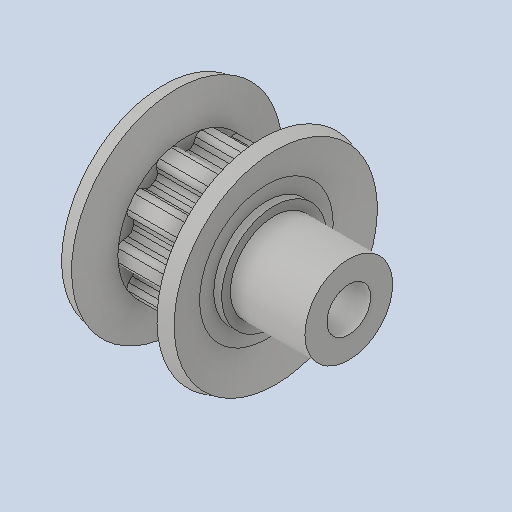
# Autodesk Inventor part: STP10XL025-B-H5_b
Saved by Autodesk Inventor 2024.1 (Build 281209000, 209)
## iProperties
Created: 2023-12-09
Part Number: STP10XL025-B-H5_b
Material: Generic
Catalog Web Link: www.cadenas.de
Description: ATP__XL025, ATP__XL031, ATP__ XL037, ATP__XL050, BTP__XL025, BTP__XL031, BTP__XL037, BTP__XL050, KTP__XL025, KTP__XL031, KTP__ XL037, KTP__XL050, NTP__XL025, NTP__XL031, NTP__ XL037, NTP__XL050, MTP__XL025, MTP__ XL037, MTP__XL050, MTPB__XL025, MTPB__ XL037, MTPB__XL050, MTPP__XL025, MTPP__ XL037, MTPP__XL050, STP__XL025, STP__XL031, STP__ XL037, STP__XL050, KATP__XL025, KATP__XL031, KATP__ XL037, KATP__XL050, KKTP__XL025, KKTP__XL031, KKTP__ XL037, KKTP__XL050_body-Timing Pulleys XL Type
Vendor: MISUMI
Document SubType Name: Modeling
Designer: psAdmin
Manufacturer: MISUMI
Mass: 3.12831 g
Surface Area: 27.7285 cm^2
Volume: 3.12831 cm^3
Density: 1 g/cm^3
Appearance: PSOLRGB-175-175-175
Category: PARTsolutions
Company: MISUMI
PSOL_IDENT_0: {$CADENAS_DATA/23d-libs/misumi/metric/51_timing_pulleys/mtp_xl/mtp_xl.prj},886 {VTYP=3D},{NB=STP10XL
PSOL_IDENT_1: 025-B-H5_b},{LINA=STP10XL025-B-H5},{NN=ATP__XL025, ATP__XL031, ATP__ XL037, ATP__XL050, BTP__XL025,
PSOL_IDENT_2: BTP__XL031, BTP__XL037, BTP__XL050, KTP__XL025, KTP__XL031, KTP__ XL037, KTP__XL050, NTP__XL025, NTP
PSOL_IDENT_3: __XL031, NTP__ XL037, NTP__XL050, MTP__XL025, MTP__ XL037, MTP__XL050, MTPB__XL025, MTPB__ XL037, MT
PSOL_IDENT_4: PB__XL050, MTPP__XL025, MTPP__ XL037, MTPP__XL050, STP__XL025, STP__XL031, STP__ XL037, STP__XL050,
PSOL_IDENT_5: KATP__XL025, KATP__XL031, KATP__ XL037, KATP__XL050, KKTP__XL025, KKTP__XL031, KKTP__ XL037, KKTP__X
PSOL_IDENT_6: L050_body},{DATE=06.01.2023 09:07:12},{GEOMDATE=06.01.2023 09:06:51},{VERSION=},{LINEID=290},{WBVAR=
PSOL_IDENT_7: MATP,ST,TNW,PS,SBS,DD,Z,J,Q,R,S,T,ALT1,ALT2,M,QSC,QFC,QTC,ALT3,K,KSC,KFC,KTC,ALT4,ZM,ZSC,ZFC,ZTC,ALT
PSOL_IDENT_8: 5,ALT6,ALT7,FC,ALT8,SRG,ALT9,BTC,TL,ALT10,TPC,ALT11,BC,ALT12,SLH,ALT13,BN},{WBNUMERIC=DD,Z,J,Q,R,S,T
PSOL_IDENT_9: ,QSC,QFC,QTC,K,KSC,KFC,KTC,ZSC,ZFC,ZTC,FC,SRG,BTC,TL,BC,SLH,BN}  {NB=STP10XL025-B-H5_b},{LINA=STP10X
PSOL_IDENT_10: L025-B-H5},{KT=DUMMY},{PN=STP10XL025-B-H5},{TYPE=STP},{MATP=SUS304},{MATPALG= 'A2017','Aluminum Allo
PSOL_IDENT_11: y 2000 series','S45C','1045 Carbon Steel Equivalent','SUS304','SUS304', 'A6000', '6000 Series Alumin
PSOL_IDENT_12: um Alloy' },{ST=-},{STALG= '-','-' },{NT=10},{TNW=XL025},{TNWALG= 'XL025','XL031','XL037','XL050' },
PSOL_IDENT_13: {BW=6.4mm (1/4inch)},{PS=B},{PSALG= 'A','B' },{SBS=H},{SBSALG= 'H','Round Hole','P','Round Hole + Ta
PSOL_IDENT_14: p','V','Stepped Hole','F','Stepped Hole (Counterbore holes on the boss side)' },{DD=5.00},{DDALG=[4:
PSOL_IDENT_15: 4/1],4.5,[5:6/1]},{DDHA=},{DDPA=},{DDNA=},{DDNK=[10:10/1]},{DDCA=},{DDVA=},{DDY=},{DDWB=},{DDHB=[4:4
PSOL_IDENT_16: /1],4.5,[5:6/1]},{DDPB=[4:4/1],4.5,[5:6/1]},{DDNB=},{DDCB=},{DDVFB=[4:4/1]},{Z=0},{ZALG=[0]},{ZMIN=7
PSOL_IDENT_17: .000},{ZAMAX=0.000},{ZBMAX=6.000},{DDZ=5.000},{J=0.0},{JALG=[0]},{JMIN=2.000},{JMAX=19.0},{JPN=},{Q=
PSOL_IDENT_18: 0},{QALG=[0]},{QRMIN=7.000},{QRMAX=8},{WBQMIN=9.000},{R=0},{RALG=[0]},{WBRMAX=-2.000},{S=0.0},{SALG=
PSOL_IDENT_19: [0]},{SMAX=6.5},{T=0.0},{TALG=[0]},{TMAX=8},{SBSPN=-H5},{A=7.5},{W=12.5},{L=21},{PD=16.17},{OD=15.66
PSOL_IDENT_20: },{D=10},{DALG=10.000},{DE=10},{F=24},{E=12},{TT=1.6},{BBK=0.000},{TTK=0.0},{ALT1=},{ANG=120.000},{A
PSOL_IDENT_21: LT1ALG= '','Not applicable' },{ALT1PN=},{ALT2=},{ALT2ALG= '','Not applicable' },{M=N/A},{MALG= 'N/A'
PSOL_IDENT_22: },{MFTALG= 'N/A' },{MSALG= 'N/A' },{M3D=0.000},{KDML=0.000},{ML=0.000},{MUL=0.000},{PITCH=0.000},{Q
PSOL_IDENT_23: SC=0.0},{QSCALG=0},{QFC=0.0},{QFCALG=0},{QTC=0.0},{QTCALG=0},{QPCDMIN=0.000},{QPCDMINALG=0.000},{QPC
PSOL_IDENT_24: DMAX=6.000},{ALT2PN=},{TAP=0.000},{ALT3=},{ALT3ALG= '','Not applicable' },{K=0.0},{KALG=0},{KMIN=4.0
PSOL_IDENT_25: 00},{KFTMAX=0.000},{KSMAX=0.000},{KSC=0.0},{KSCALG=0},{KFC=0.0},{KFCALG=0},{KTC=0.0},{KTCALG=0},{KSC
PSOL_IDENT_26: MIN=9.000},{KPCDMIN=9.000},{KPCDMAX=6.000},{ALT3PN=},{ALT4=},{ALT4ALG= '','Not applicable' },{ALT4MI
PSOL_IDENT_27: N=15.500},{ALT4MAX=1.500},{ZM=N/A},{ZMALG= 'N/A' },{ZMFTALG= 'N/A' },{ZMSALG= 'N/A' },{ZMDD1=0.0},{Z
PSOL_IDENT_28: MDD2=0.0},{ZMHH=0.0},{ZSC=0.0},{ZSCALG=[0]},{ZFC=0.0},{ZFCALG=[0]},{ZTC=0.0},{ZTCALG=[0]},{ZPCDMIN=0
PSOL_IDENT_29: .000},{ZPCDMINALG=0.000},{ZPCDMAX=6.000},{ALT4PN=},{ALT5=},{ALT5ALG= '','w/o Flange not Attached','N
PSOL_IDENT_30: FC','with NFC (Flange not Attached)' },{ALT5PN=},{ALT6=},{ALT6ALG= '','w/o Flange Attached on One Si
PSOL_IDENT_31: de Only','RFC','with RFC (Flange Attached on The Boss Side Only)','LFC','with LFC (Flange Attached o
PSOL_IDENT_32: n The Opposite Side Only)' },{ALT6PN=},{ALT7=},{ALT7ALG= '','w/o FC (Flange Cut)','FC','with FC (Fla
PSOL_IDENT_33: nge Cut)' },{FC=0.0},{FCALG=0},{FCMIN=17.0},{FCMAX=22.0},{ALT7PN=},{ALT8=},{ALT8ALG= '','Not applica
PSOL_IDENT_34: ble' },{ALT8ALGALG=6.000},{ALT8DD2=0.000},{ALT8MM=0.000},{ALT8NN=0.000},{QC=0.000},{KC=0.000},{ZC=0.
PSOL_IDENT_35: 000},{SRG=0.0},{SRGALG=[0]},{SRGMAX=0.000},{DD2=0.0},{MM=0.00},{NN=0.00},{ALT8PN=},{ALT9=},{ALT9ALG=
PSOL_IDENT_36: '','Not applicable' },{BTC9=7.000},{TL9=1.000},{BTC=0},{BTCALG=[0]},{TL=0.0},{TLALG=0},{TLMIN=1.000
PSOL_IDENT_37: },{TLMAX=-13.000},{BTCL=0},{BTCD=0},{ALT9PN=},{WLBCTL=21.000},{ALT10=},{ALT10ALG= '','Not applicable'
PSOL_IDENT_38: },{TPC=N/A},{TPCALG= 'N/A' },{TPCM=4.000},{ALT10PN=},{ALT11=},{ALT11ALG= '','w/o BC (Boss Cut)','BC'
PSOL_IDENT_39: ,'with BC (Boss Cut)' },{BC=0.0},{BCALG=0},{BCMIN=3},{BCMAX=8},{M1WBC=16},{ALT11PN=},{KTT=2.5},{ALT1
PSOL_IDENT_40: 2=},{ALT12ALG= '','Not applicable' },{SLHALG=[0]},{SLH=0},{ALT12PN=},{ALT13=},{ALT13ALG= '', 'Not ap
PSOL_IDENT_41: plicable' },{BN=0.0},{BNALG=0},{BNMIN=9},{BNMAX=18.5},{ALT13PN=},{AC=-},{M1=4.000},{M1L=3.000},{KEYA=
PSOL_IDENT_42: 0.000},{KEYB=0.000},{KEYM=0.000}
NB: STP10XL025-B-H5_b
NN: 0
NT: 10
NBSYN: $PN._b
LINA: STP10XL025-B-H5
CATALOG: Misumi
PN: STP10XL025-B-H5
MATP: SUS304
ST: -
TNW: XL025
BW: 6.4mm (1/4inch)
PS: B
SBS: Round Hole
DD: 5
Z: 0
J: 0
Q: 0
R: 0
S: 0
T: 0
A: 7.5
W: 12.5
L: 21
PD: 16.17
OD: 15.66
D: 10
F: 24
E: 12
TT: 1.6
ALT1: Not applicable
ALT2: Not applicable
M: N/A
QSC: 0
QFC: 0
QTC: 0
ALT3: Not applicable
K: 0
KSC: 0
KFC: 0
KTC: 0
ALT4: Not applicable
ZM: N/A
ZMDD1: 0
ZMDD2: 0
ZMHH: 0
ZSC: 0
ZFC: 0
ZTC: 0
ALT5: w/o Flange not Attached
ALT6: w/o Flange Attached on One Side Only
ALT7: w/o FC (Flange Cut)
FC: 0
ALT8: Not applicable
SRG: 0
DD2: 0
MM: 0
ALT9: Not applicable
BTC: 0
TL: 0
BTCL: 0
BTCD: 0
ALT10: Not applicable
TPC: N/A
ALT11: w/o BC (Boss Cut)
BC: 0
ALT12: Not applicable
SLH: 0
ALT13: Not applicable
BN: 0
AC: -
SUPPLIER: MISUMI
ARTICLENO: STP10XL025-B-H5_b
BOMINFO: STP10XL025-B-H5
CREATOR: CADENAS GmbH
Title: STP10XL025-B-H5
Author: Cadenas PARTsolutions
Comments: Timing Pulleys XL Type
Autodesk Inventor part; units mm, degrees
ref_plane "YZ Plane" through (0, 0, 0) normal (1, 0, 0) x (0, 1, 0)
ref_plane "XZ Plane" through (0, 0, 0) normal (0, 1, 0) x (-1, 0, 0)
ref_plane "XY Plane" through (0, 0, 0) normal (0, 0, 1) x (1, 0, 0)
sketch "_____3" plane through (0, 0, 0) normal (0, 0, 1) x (1, 0, 0)
  line L0 (21, 0) -> (0, 0)
  line L1 (0, 0) -> (0, 6)
  line L2 (0, 6) -> (0.9, 6)
  line L3 (0.9, 6) -> (0.9, 7.619356)
  line L4 (0.9, 7.619356) -> (-0.162829, 11.58589)
  line L5 (-0.162829, 11.58589) -> (1.382652, 12)
  line L6 (1.382652, 12) -> (2.5, 7.83)
  line L7 (2.5, 7.83) -> (10, 7.83)
  line L8 (10, 7.83) -> (11.117348, 12)
  line L9 (11.117348, 12) -> (12.662829, 11.58589)
  line L10 (12.662829, 11.58589) -> (11.6, 7.619356)
  line L11 (11.6, 7.619356) -> (11.6, 6)
  line L12 (11.6, 6) -> (12.5, 6)
  line L13 (12.5, 6) -> (12.5, 5)
  line L14 (12.5, 5) -> (21, 5)
  line L15 (21, 5) -> (21, 0)
  line L16 (21, 0) -> (0, 0)
  constraints: 34 end point
revolve "Revolution1" add sketch "_____3" angle 360 about axis through (21, 0, 0) along (1, 0, 0)
sketch "Sketch2" plane through (21, 0, 0) normal (1, 0, 0) x (0, 0, -1)
  point P0 (0, 0)
hole "Hole1" at (21, 0, 0) direction (-1, 0, 0) diameter 5 depth 21
sketch "_____6" plane through (2.5, 0, 0) normal (1, 0, 0) x (0, 0, -1)
  arc A0 (-8.085, 0) -> (-6.540902, -4.752244) centre (0, 0) ccw
  arc A1 (-6.540902, -4.752244) -> (-2.498402, -7.689292) centre (0, 0) ccw
  arc A2 (-2.498402, -7.689292) -> (2.498402, -7.689292) centre (0, 0) ccw
  arc A3 (2.498402, -7.689292) -> (6.540902, -4.752244) centre (0, 0) ccw
  arc A4 (6.540902, -4.752244) -> (8.085, 0) centre (0, 0) ccw
  arc A5 (8.085, 0) -> (6.540902, 4.752244) centre (0, 0) ccw
  arc A6 (6.540902, 4.752244) -> (2.498402, 7.689292) centre (0, 0) ccw
  arc A7 (2.498402, 7.689292) -> (-2.498402, 7.689292) centre (0, 0) ccw
  arc A8 (-2.498402, 7.689292) -> (-6.540902, 4.752244) centre (0, 0) ccw
  arc A9 (-6.540902, 4.752244) -> (-8.085, 0) centre (0, 0) ccw
  arc A10 (-7.83, 0) -> (-7.798487, -0.701787) centre (0, 0) ccw
  arc A11 (-7.798487, -0.701787) -> (-7.265282, -1.252568) centre (-7.190942, -0.647114) ccw
  line L0 (-7.265282, -1.252568) -> (-6.696552, -1.322399)
  arc A12 (-6.18421, -1.760808) -> (-6.696552, -1.322399) centre (-6.770893, -1.927852) ccw
  arc A13 (-6.18421, -1.760808) -> (-6.038108, -2.210464) centre (0, 0) ccw
  arc A14 (-6.194911, -2.866292) -> (-6.038108, -2.210464) centre (-6.61093, -2.420166) ccw
  line L1 (-6.194911, -2.866292) -> (-6.613977, -3.257077)
  arc A15 (-6.613977, -3.257077) -> (-6.721609, -4.016077) centre (-6.197958, -3.703203) ccw
  arc A16 (-6.721609, -4.016077) -> (-6.334603, -4.602359) centre (0, 0) ccw
  arc A17 (-6.334603, -4.602359) -> (-5.896608, -5.151593) centre (0, 0) ccw
  arc A18 (-5.896608, -5.151593) -> (-5.141496, -5.283774) centre (-5.43723, -4.750256) ccw
  line L2 (-5.141496, -5.283774) -> (-4.640338, -5.005978)
  arc A19 (-3.968154, -5.059511) -> (-4.640338, -5.005978) centre (-4.344604, -5.539496) ccw
  arc A20 (-3.968154, -5.059511) -> (-3.585654, -5.337414) centre (0, 0) ccw
  arc A21 (-3.327025, -5.960156) -> (-3.585654, -5.337414) centre (-3.925817, -5.843762) ccw
  line L3 (-3.327025, -5.960156) -> (-3.436358, -6.522629)
  arc A22 (-3.436358, -6.522629) -> (-3.077305, -7.199937) centre (-2.837566, -6.639023) ccw
  arc A23 (-3.077305, -7.199937) -> (-2.419603, -7.446773) centre (0, 0) ccw
  arc A24 (-2.419603, -7.446773) -> (-1.742425, -7.633666) centre (0, 0) ccw
  arc A25 (-1.742425, -7.633666) -> (-1.053833, -7.296758) centre (-1.606681, -7.038961) ccw
  line L4 (-1.053833, -7.296758) -> (-0.811672, -6.777443)
  arc A26 (-0.236398, -6.425653) -> (-0.811672, -6.777443) centre (-0.258825, -7.035241) ccw
  arc A27 (-0.236398, -6.425653) -> (0.236398, -6.425653) centre (0, 0) ccw
  arc A28 (0.811672, -6.777443) -> (0.236398, -6.425653) centre (0.258825, -7.035241) ccw
  line L5 (0.811672, -6.777443) -> (1.053833, -7.296758)
  arc A29 (1.053833, -7.296758) -> (1.742425, -7.633666) centre (1.606681, -7.038961) ccw
  arc A30 (1.742425, -7.633666) -> (2.419603, -7.446773) centre (0, 0) ccw
  arc A31 (2.419603, -7.446773) -> (3.077304, -7.199937) centre (0, 0) ccw
  arc A32 (3.077304, -7.199937) -> (3.436358, -6.522629) centre (2.837566, -6.639023) ccw
  line L6 (3.436358, -6.522629) -> (3.327025, -5.960156)
  arc A33 (3.585654, -5.337414) -> (3.327025, -5.960156) centre (3.925817, -5.843762) ccw
  arc A34 (3.585654, -5.337414) -> (3.968154, -5.059511) centre (0, 0) ccw
  arc A35 (4.640338, -5.005978) -> (3.968154, -5.059511) centre (4.344604, -5.539496) ccw
  line L7 (4.640338, -5.005978) -> (5.141496, -5.283774)
  arc A36 (5.141496, -5.283774) -> (5.896608, -5.151594) centre (5.43723, -4.750256) ccw
  arc A37 (5.896608, -5.151594) -> (6.334603, -4.602359) centre (0, 0) ccw
  arc A38 (6.334603, -4.602359) -> (6.721609, -4.016077) centre (0, 0) ccw
  arc A39 (6.721609, -4.016077) -> (6.613977, -3.257077) centre (6.197958, -3.703203) ccw
  line L8 (6.613977, -3.257077) -> (6.194911, -2.866292)
  arc A40 (6.038108, -2.210464) -> (6.194911, -2.866292) centre (6.61093, -2.420166) ccw
  arc A41 (6.038108, -2.210464) -> (6.18421, -1.760808) centre (0, 0) ccw
  arc A42 (6.696552, -1.322399) -> (6.18421, -1.760808) centre (6.770893, -1.927852) ccw
  line L9 (6.696552, -1.322399) -> (7.265282, -1.252568)
  arc A43 (7.265282, -1.252568) -> (7.798487, -0.701788) centre (7.190942, -0.647114) ccw
  arc A44 (7.798487, -0.701788) -> (7.83, 0) centre (0, 0) ccw
  arc A45 (7.83, 0) -> (7.798487, 0.701787) centre (0, 0) ccw
  arc A46 (7.798487, 0.701787) -> (7.265282, 1.252568) centre (7.190942, 0.647114) ccw
  line L10 (7.265282, 1.252568) -> (6.696552, 1.322399)
  arc A47 (6.18421, 1.760808) -> (6.696552, 1.322399) centre (6.770893, 1.927852) ccw
  arc A48 (6.18421, 1.760808) -> (6.038108, 2.210464) centre (0, 0) ccw
  arc A49 (6.194911, 2.866292) -> (6.038108, 2.210464) centre (6.61093, 2.420166) ccw
  line L11 (6.194911, 2.866292) -> (6.613977, 3.257077)
  arc A50 (6.613977, 3.257077) -> (6.721609, 4.016077) centre (6.197958, 3.703203) ccw
  arc A51 (6.721609, 4.016077) -> (6.334603, 4.602359) centre (0, 0) ccw
  arc A52 (6.334603, 4.602359) -> (5.896608, 5.151593) centre (0, 0) ccw
  arc A53 (5.896608, 5.151593) -> (5.141496, 5.283774) centre (5.43723, 4.750256) ccw
  line L12 (5.141496, 5.283774) -> (4.640338, 5.005978)
  arc A54 (3.968154, 5.059511) -> (4.640338, 5.005978) centre (4.344604, 5.539496) ccw
  arc A55 (3.968154, 5.059511) -> (3.585654, 5.337414) centre (0, 0) ccw
  arc A56 (3.327025, 5.960156) -> (3.585654, 5.337414) centre (3.925817, 5.843762) ccw
  line L13 (3.327025, 5.960156) -> (3.436358, 6.522629)
  arc A57 (3.436358, 6.522629) -> (3.077305, 7.199937) centre (2.837566, 6.639023) ccw
  arc A58 (3.077305, 7.199937) -> (2.419603, 7.446773) centre (0, 0) ccw
  arc A59 (2.419603, 7.446773) -> (1.742425, 7.633666) centre (0, 0) ccw
  arc A60 (1.742425, 7.633666) -> (1.053833, 7.296758) centre (1.606681, 7.038961) ccw
  line L14 (1.053833, 7.296758) -> (0.811672, 6.777443)
  arc A61 (0.236398, 6.425653) -> (0.811672, 6.777443) centre (0.258825, 7.035241) ccw
  arc A62 (0.236398, 6.425653) -> (-0.236398, 6.425653) centre (0, 0) ccw
  arc A63 (-0.811672, 6.777443) -> (-0.236398, 6.425653) centre (-0.258825, 7.035241) ccw
  line L15 (-0.811672, 6.777443) -> (-1.053833, 7.296758)
  arc A64 (-1.053833, 7.296758) -> (-1.742425, 7.633666) centre (-1.606681, 7.038961) ccw
  arc A65 (-1.742425, 7.633666) -> (-2.419603, 7.446773) centre (0, 0) ccw
  arc A66 (-2.419603, 7.446773) -> (-3.077304, 7.199937) centre (0, 0) ccw
  arc A67 (-3.077304, 7.199937) -> (-3.436358, 6.522629) centre (-2.837566, 6.639023) ccw
  line L16 (-3.436358, 6.522629) -> (-3.327025, 5.960156)
  arc A68 (-3.585654, 5.337414) -> (-3.327025, 5.960156) centre (-3.925817, 5.843762) ccw
  arc A69 (-3.585654, 5.337414) -> (-3.968154, 5.059511) centre (0, 0) ccw
  arc A70 (-4.640338, 5.005978) -> (-3.968154, 5.059511) centre (-4.344604, 5.539496) ccw
  line L17 (-4.640338, 5.005978) -> (-5.141496, 5.283774)
  arc A71 (-5.141496, 5.283774) -> (-5.896608, 5.151594) centre (-5.43723, 4.750256) ccw
  arc A72 (-5.896608, 5.151594) -> (-6.334603, 4.602359) centre (0, 0) ccw
  arc A73 (-6.334603, 4.602359) -> (-6.721609, 4.016077) centre (0, 0) ccw
  arc A74 (-6.721609, 4.016077) -> (-6.613977, 3.257077) centre (-6.197958, 3.703203) ccw
  line L18 (-6.613977, 3.257077) -> (-6.194911, 2.866292)
  arc A75 (-6.038108, 2.210464) -> (-6.194911, 2.866292) centre (-6.61093, 2.420166) ccw
  arc A76 (-6.038108, 2.210464) -> (-6.18421, 1.760808) centre (0, 0) ccw
  arc A77 (-6.696552, 1.322399) -> (-6.18421, 1.760808) centre (-6.770893, 1.927852) ccw
  line L19 (-6.696552, 1.322399) -> (-7.265282, 1.252568)
  arc A78 (-7.265282, 1.252568) -> (-7.798487, 0.701788) centre (-7.190942, 0.647114) ccw
  arc A79 (-7.798487, 0.701788) -> (-7.83, 0) centre (0, 0) ccw
  constraints: 160 point on circle, 80 centre point, 40 end point
extrude "Extrusion1" cut sketch "_____6" along normal blind 7.5
body "Solid1"
